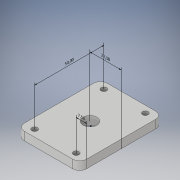
# Autodesk Inventor part: GroundToArm
Saved by Autodesk Inventor 2019 (Build 230136000, 136)
## iProperties
Created: 2018-06-10
Part Number: GroundToArm
Material: Ogólny
Document SubType Name: Modeling
Designer: Kamil
Density: 1 g/cm^3
Appearance: Domyślna
Author: Kamil
Autodesk Inventor part; units mm, degrees
ref_plane "YZ Plane" through (0, 0, 0) normal (1, 0, 0) x (0, 1, 0)
ref_plane "XZ Plane" through (0, 0, 0) normal (0, 1, 0) x (-1, 0, 0)
ref_plane "XY Plane" through (0, 0, 0) normal (0, 0, 1) x (1, 0, 0)
sketch "Szkic2" plane through (0, 0, 0) normal (0, 1, 0) x (-1, 0, 0)
  line L0 (-15, -30) -> (15, -30)
  line L1 (22.5, -25) -> (22.5, 25)
  line L2 (15, 30) -> (-15, 30)
  line L3 (-22.5, 25) -> (-22.5, -25)
  line L4 (-20, -30) -> (20, 30) construction
  line L5 (20, -30) -> (-20, 30) construction
  arc A0 (22.5, 25) -> (17.5, 30) centre (17.5, 25) ccw
  arc A1 (17.5, -30) -> (22.5, -25) centre (17.5, -25) ccw
  arc A2 (-22.5, -25) -> (-17.5, -30) centre (-17.5, -25) ccw
  arc A3 (-17.5, 30) -> (-22.5, 25) centre (-17.5, 25) ccw
  circle A4 centre (15, 25) radius 2
  circle A5 centre (15, -25) radius 2
  circle A6 centre (-15, -25) radius 2
  circle A7 centre (-15, 25) radius 2
  circle A8 centre (0, 0) radius 5
  line L6 (15, 30) -> (17.5, 30)
  line L7 (-15, 30) -> (-17.5, 30)
  line L8 (-17.5, -30) -> (-15, -30)
  line L9 (15, -30) -> (17.5, -30)
  dimension "d12" = 40
  dimension "d13" = 60
  dimension "d14" = 5
  dimension "d15" = 4
  dimension "d16" = 4
  dimension "d17" = 4
  dimension "d18" = 4
  dimension "d19" = 10
  constraints: 20 end point, 9 centre point, 8 point on circle, 5 equal length, 4 tangent, 3 equal radius, 2 horizontal, 1 coincident, 1 perpendicular
  measures "d12" distance of L5.end L4.end
  measures "d13" distance of L4.end L5.start
  measures "d14" radius of A0
  measures "d15" diameter of A4
  measures "d16" diameter of A5
  measures "d17" diameter of A6
  measures "d18" diameter of A7
  measures "d19" diameter of A8
extrude "Wyciągnięcie proste2" add sketch "Szkic2" along normal blind 6
